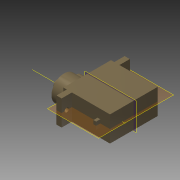
# Autodesk Inventor part: servo_metal_600TVL
Saved by Autodesk Inventor 2015 SP1 (Build 190203100, 203)
## iProperties
Created: 2015-07-09
Part Number: servo_metal_600TVL
Material: Generic
Document SubType Name: Modeling
Designer: Alexandre Cherpillod
Density: 1.75761 g/cm^3
Appearance: grey_servo
Mass: 13 g
Surface Area: 27.6353 cm^2
Volume: 7.39642 cm^3
Author: Alexandre Cherpillod
Autodesk Inventor part; units mm, degrees
ref_plane "YZ Plane" through (0, 0, 0) normal (1, 0, 0) x (0, 1, 0)
ref_plane "XZ Plane" through (0, 0, 0) normal (0, 1, 0) x (-1, 0, 0)
ref_plane "XY Plane" through (0, 0, 0) normal (0, 0, 1) x (1, 0, 0)
sketch "Sketch1" plane through (0, 0, 0) normal (0, 0, 1) x (1, 0, 0)
  line L0 (0, 0) -> (22.5, 0)
  line L1 (22.5, 0) -> (22.5, 23)
  line L2 (22.5, 23) -> (0, 23)
  line L3 (0, 23) -> (0, 0)
  dimension "d0" = 22.5
  dimension "d1" = 23
  constraints: 8 end point, 2 parallel, 1 horizontal, 1 perpendicular
  measures "d0" distance of L2.end L1.end
  measures "d1" distance of L0.end L1.end
extrude "Extrusion1" add sketch "Sketch1" along normal blind 12.2
sketch "Sketch2" plane through (0, 0, 0) normal (0, -1, 0) x (1, 0, 0)
  line L0 (0, 12.2) -> (22.5, 12.2) projected
  line L1 (0, 0) -> (22.5, 0) projected
  line L2 (1.6, 12.2) -> (4.1, 12.2)
  line L3 (4.1, 12.2) -> (4.1, 0)
  line L4 (4.1, 0) -> (1.6, 0)
  line L5 (1.6, 0) -> (1.6, 12.2)
  line L6 (22.5, 0) -> (22.5, 12.2) projected
  dimension "d4" = 2.5
  dimension "d5" = 18.4
  constraints: 8 end point, 2 parallel, 2 point on line, 1 horizontal, 1 perpendicular
  measures "d4" distance between parallel lines of L3 L5
  measures "d5" distance between parallel lines of L6 L3
extrude "Extrusion2" add sketch "Sketch2" along normal blind 5 contours L0 L3 L1 L5
ref_plane "Work Plane1" through (22.5, 11.5, 0) normal (0, -1, 0) x (1, 0, 0)
mirror "Mirror1" about plane through (22.5, 11.5, 0) normal (0, -1, 0) of "Extrusion2"
ref_plane "Work Plane3" through (0, -2.5, 0) normal (0, -1, 0) x (1, 0, 0)
ref_plane "Work Plane4" through (0, 0, 6.1) normal (0, 0, 1) x (1, 0, 0)
hole "Hole1" at (1.6, -2.5, 6.1) direction (1, 0, 0) diameter 2 end through all
mirror "Mirror2" about plane through (22.5, 11.5, 0) normal (0, -1, 0) of "Hole1"
sketch "Sketch3" plane through (22.5, 0, 0) normal (0, -1, 0) x (1, 0, 0)
  line L0 (-4.7, 4.35) -> (-6, 4.35)
  line L1 (-6, 4.35) -> (-6, 7.85)
  line L2 (-6, 7.85) -> (-4.7, 7.85)
  line L3 (-4.7, 7.85) -> (-4.7, 4.35)
  line L4 (0, 12.2) -> (0, 0) projected
  line L5 (0, 0) -> (-18.4, 0) projected
  line L6 (-18.4, 12.2) -> (-18.4, 0) projected
  line L7 (-20.9, 12.2) -> (-18.4, 12.2) projected
  line L8 (-20.9, 0) -> (-20.9, 12.2) projected
  line L9 (-20.9, 0) -> (-22.5, 0) projected
  line L10 (-22.5, 0) -> (-22.5, 12.2) projected
  line L11 (-22.5, 12.2) -> (-20.9, 12.2) projected
  line L12 (-18.4, 12.2) -> (0, 12.2) projected
  line L13 (-18.4, 0) -> (-20.9, 0) projected
  line L14 (0, 12.2) -> (0, 0) projected
  line L15 (0, 0) -> (-18.4, 0) projected
  line L16 (-18.4, 12.2) -> (-18.4, 0) projected
  line L17 (-20.9, 12.2) -> (-18.4, 12.2) projected
  line L18 (-20.9, 0) -> (-20.9, 12.2) projected
  line L19 (-20.9, 0) -> (-22.5, 0) projected
  line L20 (-22.5, 0) -> (-22.5, 12.2) projected
  line L21 (-22.5, 12.2) -> (-20.9, 12.2) projected
  line L22 (-18.4, 12.2) -> (0, 12.2) projected
  line L23 (-18.4, 0) -> (-20.9, 0) projected
  line L24 (0, 12.2) -> (0, 0) projected
  line L25 (0, 0) -> (-18.4, 0) projected
  line L26 (-18.4, 12.2) -> (-18.4, 0) projected
  line L27 (-20.9, 12.2) -> (-18.4, 12.2) projected
  line L28 (-20.9, 0) -> (-20.9, 12.2) projected
  line L29 (-20.9, 0) -> (-22.5, 0) projected
  line L30 (-22.5, 0) -> (-22.5, 12.2) projected
  line L31 (-22.5, 12.2) -> (-20.9, 12.2) projected
  line L32 (-18.4, 12.2) -> (0, 12.2) projected
  line L33 (-18.4, 0) -> (-20.9, 0) projected
  line L34 (-27, 6.1) -> (4.5, 6.1) projected
  point P0 (-6, 6.1)
  dimension "d17" = 1.3
  dimension "d18" = 3.5
  dimension "d19" = 4.7
  constraints: 8 end point, 2 parallel, 1 horizontal, 1 midpoint, 1 perpendicular, 1 point on line
  measures "d17" distance of L1.end L2.end
  measures "d18" distance of L0.end L1.end
  measures "d19" distance between parallel lines of L14 L3
extrude "Extrusion3" add sketch "Sketch3" along normal blind 2 contours L0 L1 L34 L3 | L34 L1 L2 L3
sketch "Sketch4" plane through (0, 0, 0) normal (-1, 0, 0) x (0, 0, 1)
  line L0 (6.1, 34.6) -> (6.1, -11.6) projected
  circle A0 centre (6.1, 6.1) radius 6.1
  line L1 (0, 0) -> (0, 23) projected
  line L2 (0, 0) -> (12.2, 0) projected
  constraints: 2 tangent, 1 centre point, 1 point on line
extrude "Extrusion4" add sketch "Sketch4" along normal blind 5.8 contours A0 L0 | L0 A0
sketch "Sketch5" plane through (-5.8, 6.1, 6.1) normal (-1, 0, 0) x (0, 0, 1)
  circle A0 centre (0, 0) radius 2
  point P0 (-6.1, -6.1)
  dimension "d24" = 4
  constraints: 1 centre point
  measures "d24" diameter of A0
extrude "Extrusion5" add sketch "Sketch5" along normal blind 3.25
sketch "Sketch6" plane through (0, 23, 0) normal (-1, 0, 0) x (0, 0, 1)
  circle A0 centre (6.1, -16.9) radius 6.1 projected
  arc A1 (12.2, -16.9) -> (0, -16.9) centre (6.1, -16.9) ccw projected
  circle A2 centre (6.1854, -10.8006) radius 2.5717
  point P0 (0, -23)
  constraints: 2 point on circle, 1 centre point
extrude "Extrusion6" add sketch "Sketch6" along normal up to surface (5.8 mm away) contours A2 A0 | A0 A2 picked at (5.289, -10.1215) picked at (6.9125, -11.6556)
ref_plane "Work Plane2" through (22.5, 11.5, 0) normal (0, -1, 0) x (1, 0, 0)
body "Solid1"
